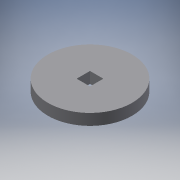
# Autodesk Inventor part: sensor wheel
Saved by Autodesk Inventor 2017 SP1 (Build 210196100, 196)
## iProperties
Created: 2017-06-15
Part Number: sensor wheel
Material: Generic
Document SubType Name: Modeling
Designer: RMcComber
Density: 1 g/cm^3
Appearance: Default
Author: RMcComber
Autodesk Inventor part; units mm, degrees
ref_plane "YZ Plane" through (0, 0, 0) normal (1, 0, 0) x (0, 1, 0)
ref_plane "XZ Plane" through (0, 0, 0) normal (0, 1, 0) x (-1, 0, 0)
sketch "Sketch1" plane through (0, 0, 0) normal (0, 0, 1) x (1, 0, 0)
  circle A0 centre (0, 0) radius 30
  line L0 (4.7625, -4.7625) -> (-4.7625, -4.7625)
  line L1 (-4.7625, -4.7625) -> (-4.7625, 4.7625)
  line L2 (-4.7625, 4.7625) -> (4.7625, 4.7625)
  line L3 (4.7625, 4.7625) -> (4.7625, -4.7625)
  line L4 (4.7625, -4.7625) -> (-4.7625, 4.7625) construction
  line L5 (-4.7625, -4.7625) -> (4.7625, 4.7625) construction
  dimension "d0" = 60
  dimension "d15" = 9.525
  constraints: 12 end point, 2 midpoint, 2 parallel, 2 perpendicular, 1 centre point, 1 coincident, 1 horizontal
  measures "d0" diameter of A0
  measures "d15" distance of L1.end L2.end
extrude "Extrusion1" add sketch "Sketch1" along normal blind 8
sketch "Sketch2" plane through (0, 0, 8) normal (0, 0, 1) x (1, 0, 0)
  circle A0 centre (0, 0) radius 30 projected
  line L0 (0, 0) -> (0, 25) construction
  circle A1 centre (0, 25) radius 3
  dimension "d4" = 6
  dimension "d5" = 25
  constraints: 2 end point, 1 centre point, 1 coincident, 1 vertical
  measures "d4" diameter of A1
  measures "d5" distance of L0.start L0.end
extrude "Extrusion2" [suppressed]
sketch "Sketch3" plane through (0, 0, 0) normal (0, 0, -1) x (-1, 0, 0)
  line L0 (-4.7625, 0) -> (-12.5, 0)
  line L1 (-12.5, 0) -> (-12.5, -10)
  line L2 (-12.5, -10) -> (12.5, -10)
  line L3 (12.5, -10) -> (12.5, 0)
  line L4 (12.5, 0) -> (4.7625, 0)
  line L5 (4.7625, 4.7625) -> (4.7625, -4.7625) construction
  line L6 (-4.7625, -4.7625) -> (-4.7625, 4.7625) construction
  line L7 (4.7625, -4.7625) -> (-4.7625, -4.7625) construction
  line L8 (4.7625, -4.7625) -> (4.7625, 4.7625) projected
  line L9 (4.7625, 0) -> (4.7625, -4.7625)
  line L10 (4.7625, -4.7625) -> (-4.7625, -4.7625)
  line L11 (-4.7625, 4.7625) -> (-4.7625, -4.7625) projected
  line L12 (-4.7625, -4.7625) -> (-4.7625, 0)
  dimension "d8" = 10
  dimension "d9" = 25
  constraints: 16 end point, 5 collinear, 2 midpoint, 2 parallel, 2 perpendicular, 1 horizontal
  measures "d8" distance of L0.end L1.end
  measures "d9" distance of L1.end L2.end
extrude "Extrusion3" add sketch "Sketch3" along normal blind 6
sketch "Sketch4" plane through (-12.5, 0, 0) normal (0, 1, 0) x (1, 0, 0)
  line L0 (21.1313, 6) -> (21.1313, 0) construction
  line L1 (3.8687, 6) -> (3.8687, 0) construction
  circle A0 centre (21.1312, 3) radius 1.4
  circle A1 centre (3.8687, 3) radius 1.4
  line L2 (7.7375, 0) -> (0, 0) construction
  line L3 (7.7375, 0) -> (7.7375, 6) construction
  line L4 (0, 6) -> (7.7375, 6) construction
  line L5 (0, 0) -> (0, 6) construction
  line L6 (25, 0) -> (17.2625, 0) construction
  line L7 (25, 0) -> (25, 6) construction
  line L8 (17.2625, 6) -> (25, 6) construction
  line L9 (17.2625, 0) -> (17.2625, 6) construction
  line L10 (0, 6) -> (7.7375, 6) construction
  line L11 (7.7375, 0) -> (0, 0) construction
  line L12 (17.2625, 6) -> (25, 6) construction
  dimension "d12" = 2.8
  constraints: 6 midpoint, 4 end point, 2 centre point, 1 equal radius
  measures "d12" diameter of A0
extrude "Extrusion4" cut sketch "Sketch4" against normal through all
ref_plane "Work Plane1" through (0, 30, 0) normal (0, 1, 0) x (-1, 0, 0)
sketch "Sketch5" plane through (0, 30, 0) normal (0, 1, 0) x (-1, 0, 0)
  line L0 (30, 8) -> (-30, 8) construction
  line L1 (-30, 0) -> (30, 0) construction
  line L2 (30, 8) -> (-30, 8) construction
  line L3 (0, 8) -> (0, 0) construction
  circle A0 centre (0, 4) radius 3
  dimension "d16" = 6
  constraints: 2 end point, 2 midpoint, 1 centre point, 1 vertical
  measures "d16" diameter of A0
extrude "Extrusion5" cut sketch "Sketch5" against normal blind 4
body "Solid1"
